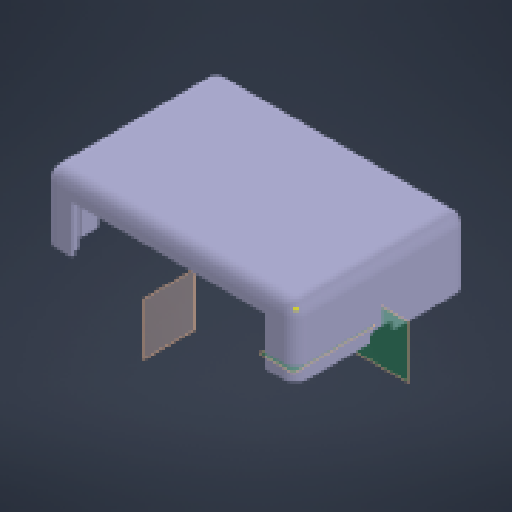
# Autodesk Inventor part: case2
Saved by Autodesk Inventor 2025.2 (Build 292293000, 293)
## iProperties
Created: 2025-10-05
Part Number: case2
Material: Generic
Document SubType Name: Modeling
Designer: micyg
Density: 1 g/cm^3
Appearance: Default
Author: micyg
Autodesk Inventor part; units mm, degrees
ref_plane "YZ Plane" through (0, 0, 0) normal (1, 0, 0) x (0, 1, 0)
ref_plane "XZ Plane" through (0, 0, 0) normal (0, 1, 0) x (-1, 0, 0)
ref_plane "XY Plane" through (0, 0, 0) normal (0, 0, 1) x (1, 0, 0)
sketch "Sketch1" plane through (0, 0, 0) normal (0, 1, 0) x (-1, 0, 0)
  line L0 (0, 0) -> (105, 0)
  line L1 (105, 0) -> (105, -72)
  line L2 (105, -72) -> (0, -72)
  line L3 (0, -72) -> (0, 0)
  dimension "d0" = 105
  dimension "d1" = 72
  constraints: 8 end point, 2 parallel, 1 horizontal, 1 perpendicular
  measures "d0" distance of L1.end L2.end
  measures "d1" distance of L0.end L1.end
extrude "Extrusion1" add sketch "Sketch1" along normal blind 28
fillet "Fillet1" radius 5 4 edges at (-105, 14, 0) (0, 14, 0) (-105, 14, -72) (0, 14, -72)
fillet "Fillet2" radius 5 8 edges at (-1.4645, 28, -70.5355) (-52.5, 28, -72) (-103.5355, 28, -70.5355) (-105, 28, -36) (-103.5355, 28, -1.4645) (-52.5, 28, 0) (-1.4645, 28, -1.4645) (0, 28, -36)
shell "Shell2" thickness 3 removed faces 1 at (-36.6667, 0, -48)
sketch "Sketch2" plane through (0, 0, 0) normal (0, -1, 0) x (1, 0, 0)
  arc A0 (-5, -69) -> (-3, -67) centre (-5, -67) ccw projected
  line L0 (-5, -69) -> (-100, -69) projected
  arc A1 (-102, -67) -> (-100, -69) centre (-100, -67) ccw projected
  line L1 (-102, -67) -> (-102, -5) projected
  arc A2 (-100, -3) -> (-102, -5) centre (-100, -5) ccw projected
  line L2 (-100, -3) -> (-5, -3) projected
  arc A3 (-3, -5) -> (-5, -3) centre (-5, -5) ccw projected
  line L3 (-3, -5) -> (-3, -67) projected
  arc A4 (-5, -72) -> (0, -67) centre (-5, -67) ccw projected
  line L4 (0, -5) -> (0, -67) projected
  arc A5 (0, -5) -> (-5, 0) centre (-5, -5) ccw projected
  line L5 (-100, 0) -> (-5, 0) projected
  arc A6 (-100, 0) -> (-105, -5) centre (-100, -5) ccw projected
  line L6 (-105, -67) -> (-105, -5) projected
  arc A7 (-105, -67) -> (-100, -72) centre (-100, -67) ccw projected
  line L7 (-5, -72) -> (-100, -72) projected
  arc A8 (-5, -70.6) -> (-1.4, -67) centre (-5, -67) ccw
  line L8 (-5, -70.6) -> (-100, -70.6)
  arc A9 (-103.6, -67) -> (-100, -70.6) centre (-100, -67) ccw
  line L9 (-103.6, -67) -> (-103.6, -5)
  arc A10 (-100, -1.4) -> (-103.6, -5) centre (-100, -5) ccw
  line L10 (-100, -1.4) -> (-5, -1.4)
  arc A11 (-1.4, -5) -> (-5, -1.4) centre (-5, -5) ccw
  line L11 (-1.4, -5) -> (-1.4, -67)
  point P0 (0, 0)
  dimension "d8" = 1.4
  constraints: 8 end point, 8 point on circle, 4 centre point, 7 other
  measures "d8" distance between parallel lines of L4 L11
extrude "Extrusion2" cut sketch "Sketch2" against normal blind 1.6 contours L8 A9 L9 A10 L10 A11 L11 A8
sketch "Sketch3" plane through (-102, 23, -5) normal (1, 0, 0) x (0, 0, -1)
  line L0 (41.5, -23.005) -> (41.5, -3.505) projected
  line L1 (22, -23.005) -> (41.5, -23.005) projected
  line L2 (22, -23.005) -> (22, -3.505) projected
  line L3 (41.5, -3.505) -> (22, -3.505) projected
  circle A0 centre (31, -13.005) radius 7 projected
  line L4 (62, -23) -> (65.6, -23) projected
  line L5 (65.6, -23) -> (62, -23) projected
  line L6 (62, -23) -> (0, -23) projected
  line L7 (0, -23) -> (-3.6, -23) projected
  line L8 (-3.6, -23) -> (0, -23) projected
  line L9 (0, -23) -> (62, -23) projected
  line L10 (62, -23) -> (67, -23) projected
  line L11 (0, -23) -> (62, -23) projected
  line L12 (-5, -23) -> (0, -23) projected
  line L13 (0, -23) -> (-5, -23) projected
  line L14 (62, -23) -> (0, -23) projected
  line L15 (67, -23) -> (62, -23) projected
  line L16 (42, -3.005) -> (42, -23.505)
  line L17 (42, -23.505) -> (21.5, -23.505)
  line L18 (21.5, -23.505) -> (21.5, -3.005)
  line L19 (21.5, -3.005) -> (42, -3.005)
  dimension "d11" = 0.5
  constraints: 8 end point, 3 other
  measures "d11" distance between parallel lines of L0 L16
extrude "Extrusion3" cut sketch "Sketch3" against normal up to surface (3 mm away) contours L1 L2 L6 L0 | L0 L6 L16 L17 L18 L2 L1 | L6 L2 L3 L0 | L0 L3 L2 L6 L18 L19 L16 | A0
sketch "Sketch4" plane through (-100, 23, -69) normal (0, 0, 1) x (1, 0, 0)
  line L0 (67, -23.005) -> (67, -3.505) projected
  line L1 (86.5, -23.005) -> (67, -23.005) projected
  line L2 (86.5, -23.005) -> (86.5, -3.505) projected
  line L3 (67, -3.505) -> (86.5, -3.505) projected
  circle A0 centre (77.5, -13.005) radius 7 projected
  line L4 (47, -23.005) -> (47, -3.505) projected
  line L5 (66.5, -23.005) -> (47, -23.005) projected
  line L6 (66.5, -23.005) -> (66.5, -3.505) projected
  line L7 (47, -3.505) -> (66.5, -3.505) projected
  circle A1 centre (57.5, -13.005) radius 7 projected
  line L8 (27, -23.005) -> (27, -3.505) projected
  line L9 (46.5, -23.005) -> (27, -23.005) projected
  line L10 (46.5, -23.005) -> (46.5, -3.505) projected
  line L11 (27, -3.505) -> (46.5, -3.505) projected
  circle A2 centre (37.5, -13.005) radius 7 projected
  line L12 (7, -23.005) -> (7, -3.505) projected
  line L13 (26.5, -23.005) -> (7, -23.005) projected
  line L14 (26.5, -23.005) -> (26.5, -3.505) projected
  line L15 (7, -3.505) -> (26.5, -3.505) projected
  circle A3 centre (17.5, -13.005) radius 7 projected
  line L16 (87, -3.005) -> (6.5, -3.005)
  line L17 (6.5, -3.005) -> (6.5, -23.505)
  line L18 (6.5, -23.505) -> (87, -23.505)
  line L19 (87, -23.505) -> (87, -3.005)
  point P0 (100, -23)
  dimension "d14" = 0.5
  dimension "d15" = 0.5
  dimension "d16" = 0.5
  dimension "d17" = 0.5
  constraints: 8 end point, 2 parallel, 1 horizontal, 1 perpendicular
  measures "d14" distance between parallel lines of L12 L17
  measures "d15" distance between parallel lines of L18 L13
  measures "d16" distance between parallel lines of L16 L15
  measures "d17" distance between parallel lines of L19 L2
extrude "Extrusion4" cut sketch "Sketch4" against normal up to surface (3 mm away) contours L0 L3 L2 L1 | A0 | L4 L7 L6 L5 | A1 | L8 L11 L10 L9 | A2 | L12 L15 L14 L13 | A3 | L19 L18 L17 L16
ref_plane "Work Plane2" through (-52.5, 0, 0) normal (1, 0, 0) x (0, 1, 0)
ref_plane "Work Plane3" through (0, 0, -36) normal (0, 0, -1) x (-1, 0, 0)
mirror "Mirror1" about plane through (0, 0, -36) normal (0, 0, -1) of "Extrusion4"
sketch "Sketch6" plane through (0, 0, -5) normal (1, 0, 0) x (0, 0, -1)
  line L0 (31, 0.345) -> (31, 0.145) construction
  line L1 (27.81, 0.345) -> (31, 0.345) construction
  arc A0 (26.73, 1.425) -> (27.81, 0.345) centre (27.81, 1.425) ccw construction
  line L2 (26.73, 2.025) -> (26.73, 1.425) construction
  arc A1 (27.81, 3.105) -> (26.73, 2.025) centre (27.81, 2.025) ccw construction
  line L3 (31, 3.105) -> (27.81, 3.105) construction
  line L4 (31, 3.305) -> (31, 3.105) construction
  line L5 (31, 3.305) -> (27.81, 3.305) construction
  arc A2 (27.81, 3.305) -> (26.53, 2.025) centre (27.81, 2.025) ccw construction
  line L6 (26.53, 2.025) -> (26.53, 1.425) construction
  arc A3 (26.53, 1.425) -> (27.81, 0.145) centre (27.81, 1.425) ccw construction
  line L7 (27.81, 0.145) -> (31, 0.145) construction
  line L8 (31, 0.345) -> (31, 0.145) construction
  line L9 (34.19, 0.145) -> (31, 0.145) construction
  arc A4 (34.19, 0.145) -> (35.47, 1.425) centre (34.19, 1.425) ccw construction
  line L10 (35.47, 2.025) -> (35.47, 1.425) construction
  arc A5 (35.47, 2.025) -> (34.19, 3.305) centre (34.19, 2.025) ccw construction
  line L11 (31, 3.305) -> (34.19, 3.305) construction
  line L12 (31, 3.305) -> (31, 3.105) construction
  line L13 (31, 3.105) -> (34.19, 3.105) construction
  arc A6 (35.27, 2.025) -> (34.19, 3.105) centre (34.19, 2.025) ccw construction
  line L14 (35.27, 2.025) -> (35.27, 1.425) construction
  arc A7 (34.19, 0.345) -> (35.27, 1.425) centre (34.19, 1.425) ccw construction
  line L15 (34.19, 0.345) -> (31, 0.345) construction
  line L16 (31, 3.805) -> (27.81, 3.805)
  arc A8 (27.81, 3.805) -> (26.03, 2.025) centre (27.81, 2.025) ccw
  line L17 (26.03, 2.025) -> (26.03, 1.425)
  arc A9 (26.03, 1.425) -> (27.81, -0.355) centre (27.81, 1.425) ccw construction
  line L18 (27.81, -0.355) -> (31, -0.355)
  line L19 (31, 3.805) -> (34.19, 3.805)
  arc A10 (35.97, 2.025) -> (34.19, 3.805) centre (34.19, 2.025) ccw
  line L20 (35.97, 2.025) -> (35.97, 1.425)
  arc A11 (34.19, -0.355) -> (35.97, 1.425) centre (34.19, 1.425) ccw construction
  line L21 (34.19, -0.355) -> (31, -0.355)
  line L22 (0, 23) -> (62, 23) construction
  line L23 (0, 0) -> (0, 23) construction
  line L24 (0, 0) -> (62, 0) construction
  line L25 (62, 23) -> (62, 0) construction
  line L26 (35.97, 3.805) -> (26.03, 3.805)
  line L27 (26.03, 3.805) -> (26.03, -0.355)
  line L28 (26.03, -0.355) -> (35.97, -0.355)
  line L29 (35.97, -0.355) -> (35.97, 3.805)
  point P0 (-5, 0)
  dimension "d23" = 0.5
  constraints: 20 end point, 8 point on circle, 4 centre point, 4 point on line, 2 parallel, 1 horizontal, 1 perpendicular, 8 other
  measures "d23" distance between parallel lines of L7 L18
extrude "Extrusion6" cut sketch "Sketch6" against normal up to surface (3 mm away) contours L19 A10 L20 L29 L28 L21 L18 L27 L17 A8 L16
ref_plane "Work Plane4" through (0, 6, 0) normal (0, -1, 0) x (1, 0, 0)
sketch "Sketch9" plane through (0, 6, 0) normal (0, -1, 0) x (1, 0, 0)
  line L0 (-3, -31.03) -> (-1.4, -31.03) projected
  line L1 (-1.4, -5) -> (-1.4, -31.03) projected
  arc A0 (-1.4, -5) -> (-5, -1.4) centre (-5, -5) ccw projected
  line L2 (-13, -1.4) -> (-5, -1.4) projected
  line L3 (-13, -1.4) -> (-13, -3) projected
  line L4 (-5, -3) -> (-13, -3) projected
  arc A1 (-3, -5) -> (-5, -3) centre (-5, -5) ccw projected
  line L5 (-3, -31.03) -> (-3, -5) projected
  arc A2 (-12.5, -8.5) -> (-8.5, -12.5) centre (-8.5, -8.5) ccw
  line L6 (-8.5, -12.5) -> (-3, -12.5)
  line L7 (-12.5, -3) -> (-12.5, -8.5)
  line L8 (-52.5, 14.4) -> (-52.5, -86.4) projected
  line L9 (21, -36) -> (-126, -36) projected
  line L10 (-96.5, -8.5) -> (-8.5, -8.5) construction
  line L11 (-8.5, -8.5) -> (-8.5, -63.5) construction
  line L12 (-8.5, -63.5) -> (-96.5, -63.5) construction
  line L13 (-96.5, -63.5) -> (-96.5, -8.5) construction
  line L14 (-96.5, -8.5) -> (-8.5, -63.5) construction
  line L15 (-8.5, -8.5) -> (-96.5, -63.5) construction
  circle A3 centre (-8.5, -8.5) radius 1.5
  point P0 (0, 0)
  point P1 (-52.5, -36)
  dimension "d28" = 88
  dimension "d29" = 55
  dimension "d30" = 3
  dimension "d31" = 2.5
  constraints: 16 end point, 4 midpoint, 4 point on line, 2 centre point, 2 coincident, 2 parallel, 2 perpendicular, 2 point on circle, 2 tangent, 1 horizontal, 1 vertical
  measures "d28" distance of L11.end L12.end
  measures "d29" distance of L10.end L11.end
  measures "d30" diameter of A3
  measures "d31" radial gap between concentric circles of A2 A3
extrude "Extrusion7" add sketch "Sketch9" against normal up to surface (19 mm away) contours L6 A2 L7 L4 A1 L5
mirror "Mirror2" about plane through (0, 0, -36) normal (0, 0, -1) of "Extrusion7"
mirror "Mirror3" about plane through (-52.5, 0, 0) normal (1, 0, 0) of "Extrusion7", "Mirror2"
sketch "Sketch10" plane through (0, 28, 0) normal (0, 1, 0) x (1, 0, 0)
  point P0 (0, 0)
equation "\"d6\" = d5"
equation "\"d15\" = d14"
equation "\"d16\" = d14"
equation "\"d17\" = d14"
equation "\"d5\" = 5"
body "Solid1"
